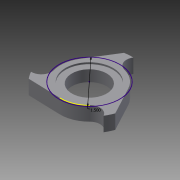
# Autodesk Inventor part: Spinner 1
Saved by Autodesk Inventor 2018 (Build 220112000, 112)
## iProperties
Created: 2017-12-13
Part Number: Spinner 1
Material: Generic
Document SubType Name: Modeling
Designer: Rus
Density: 1 g/cm^3
Appearance: Default
Author: Rus
Autodesk Inventor part; units mm, degrees
ref_plane "YZ Plane" through (0, 0, 0) normal (1, 0, 0) x (0, 1, 0)
sketch "Sketch3" plane through (0, 0, 0) normal (1, 0, 0) x (0, 1, 0)
  line L0 (0, 0) -> (0, -11) construction
  line L1 (0, 0) -> (7, 0) construction
  line L2 (7, 0) -> (7, -11) construction
  line L3 (0, -11) -> (0, -41.91)
  line L4 (0, -41.91) -> (-1.9706, -41.91) construction
  line L5 (0, -11) -> (7, -11)
  line L6 (7, -11) -> (7, -41.91)
  line L7 (0, -41.91) -> (0, -39.6842) construction
  line L8 (0, -41.91) -> (7, -41.91)
  dimension "d7" = 7
  dimension "d8" = 11
  dimension "d9" = 41.91
  constraints: 18 end point, 4 horizontal, 2 perpendicular, 2 vertical, 1 parallel, 1 point on line
  measures "d7" distance of L0.start L1.end
  measures "d8" distance of L1.end L2.end
  measures "d9" distance from line of L3.end L1
revolve "Revolution1" add sketch "Sketch3" angle 360 about axis through (0, 0, 0) along (0, 1, 0)
ref_plane "Work Plane2" through (0, 0, 0) normal (-1, 0, 0) x (0, 1, 0)
sketch "Sketch4" plane through (0, 0, 0) normal (-1, 0, 0) x (0, 1, 0)
  line L0 (0, 0) -> (7, 0)
  line L1 (7, 41.91) -> (7, -41.91) projected
  line L2 (7, 0) -> (7, 11)
  line L3 (7, 0) -> (8, 0)
  line L4 (8, 0) -> (8, 15)
  line L5 (8, 15) -> (7, 15)
  line L6 (8, 15) -> (8, 41.91)
  line L7 (8, 41.91) -> (7, 41.91)
  line L8 (0, 0) -> (0, 0.75)
  line L9 (0, 11) -> (0, -11) projected
  line L10 (8, 15) -> (0, 15)
  line L11 (0, 41.91) -> (0, -41.91) projected
  line L12 (0, 15) -> (-1, 15)
  line L13 (-1, 15) -> (-1, 41.91)
  line L14 (-1, 41.91) -> (0, 41.91)
  dimension "d16" = 11
  dimension "d17" = 1
  dimension "d18" = 15
  dimension "d20" = 0.75
  dimension "d21" = 1
  constraints: 24 end point, 4 horizontal, 3 perpendicular, 3 point on line, 2 vertical, 1 midpoint, 1 parallel
  measures "d16" distance of L0.end L2.end
  measures "d17" distance of L0.end L3.end
  measures "d18" distance of L3.end L4.end
  measures "d20" distance of L0.start L8.end
  measures "d21" distance of L10.end L12.end
ref_plane "Work Plane3" through (0, 3.5, 0) normal (0, 1, 0) x (1, 0, 0)
revolve "Revolution2" add sketch "Sketch4" angle 360 about axis through (0, 0, 0) along (0, 1, 0) contours L12 L13 L14 L11 | L1 L7 L6 L5
sketch "Sketch5" plane through (0, 8, 0) normal (0, 1, 0) x (1, 0, 0)
  circle A0 centre (0, 0) radius 18.175
  circle A1 centre (0, 0) radius 15 projected
  circle A2 centre (0, 0) radius 41.91 projected
  circle A3 centre (0, 0) radius 35.56
  dimension "d22" = 3.175
  dimension "d23" = 6.35
  constraints: 2 centre point, 2 coincident
  measures "d22" radial gap between concentric circles of A0 A1
  measures "d23" radial gap between concentric circles of A2 A3
extrude "Extrusion2" cut sketch "Sketch5" against normal through all contours A3
sketch "Sketch6" plane through (0, 8, 0) normal (0, 1, 0) x (1, 0, 0)
  circle A0 centre (0, 0) radius 18.175 projected
  circle A1 centre (0, 0) radius 35.56 projected
  line L0 (16.0245, 8.5759) -> (30.4464, -18.372)
  line L1 (27.5834, -22.4426) -> (17.7246, -4.0211)
  dimension "d26" = 4.445
  constraints: 4 end point, 4 point on circle, 1 parallel, 1 tangent
  measures "d26" distance between parallel lines of L1 L0
extrude "Extrusion3" add sketch "Sketch6" against normal up to surface (9 mm away) contours A0 L0 A1 L1 picked at (22.1844, -5.1361)
pattern_circular "Circular Pattern1" count 3 over 360 about axis through (0, 3.5, 0) along (0, -1, 0) of "Extrusion3"
fillet "Fillet1" radius 6.35 3 edges at (-5.3799, 3.5, -17.3605) (17.7246, 3.5, 4.0211) (-12.3447, 3.5, 13.3394)
fillet "Fillet1" radius 3.175 3 edges at (27.5834, 3.5, 22.4426) (-33.2276, 3.5, 12.6666) (5.6442, 3.5, -35.1092)
fillet "Fillet1" radius 3.175 3 edges at (0.6874, 3.5, -35.5534) (-31.1338, 3.5, 17.1814) (30.4464, 3.5, 18.372)
sketch "Sketch7" plane through (0, 0, 0) normal (-1, 0, 0) x (0, 1, 0)
  line L0 (8, -41.91) -> (8, 41.91) projected
  line L1 (-1, -41.91) -> (-1, 41.91) projected
  line L2 (8, -41.91) -> (-1, -41.91) projected
  arc A0 (6.04, -41.91) -> (8, -35.56) centre (-3.2664, -35.56) ccw
  arc A1 (-1, -35.56) -> (0.96, -41.91) centre (10.2664, -35.56) ccw
  line L3 (0.96, -41.91) -> (6.04, -41.91)
  line L4 (-1, -35.56) -> (8, -35.56)
  line L5 (8, -22.57) -> (-1, -22.57) projected
  line L6 (8, -24.1718) -> (8, -35.56) projected
  line L7 (-1, -24.1718) -> (8, -24.1718) projected
  line L8 (-1, -22.57) -> (-1, -24.1718) projected
  line L9 (8, -35.56) -> (8, -35.56) projected
  line L10 (0, 0) -> (11.7377, 0)
  dimension "d36" = 6.35
  dimension "d37" = 5.08
  constraints: 6 end point, 4 point on circle, 4 point on line, 2 centre point, 2 horizontal, 2 tangent, 1 collinear, 1 equal radius, 1 midpoint
  measures "d36" distance between parallel lines of L2 L4
  measures "d37" distance of L3.end L3.start
revolve "Revolution3" cut sketch "Sketch7" angle 360 about axis through (0, 0, 0) along (0, 1, 0) contours L2 A0 L0 | A1 L2 L1
fillet "Fillet2" radius 1.5875 4 edges at (41.91, 6.04, 0) (-41.91, 6.04, 0) (-41.91, 0.96, 0) (41.91, 0.96, 0)
sketch "Sketch8" plane through (27.5145, 8, 12.8937) normal (0, 1, 0) x (0.8816766, 0, -0.4718541)
  circle A0 centre (-18.175, 24.3509) radius 19.05
  arc A1 (-27.2625, 8.6109) -> (-12.7058, 7.0183) centre (-18.175, 24.3509) ccw projected
  dimension "d40" = 38.1
  constraints: 1 centre point, 1 coincident
  measures "d40" diameter of A0
sketch "Sketch9" plane through (27.5145, 8, 12.8937) normal (0, 1, 0) x (0.8816766, 0, -0.4718541)
  circle A0 centre (-18.175, 24.3509) radius 27.1145
  circle A1 centre (-18.175, 24.3509) radius 41.91
  circle A2 centre (-18.175, 24.3509) radius 41.91 projected
  dimension "d41" = 54.229
  constraints: 2 centre point, 2 coincident, 1 concentric
  measures "d41" diameter of A0
extrude "Extrusion4" cut sketch "Sketch9" against normal blind 25.4
body "Solid2"
